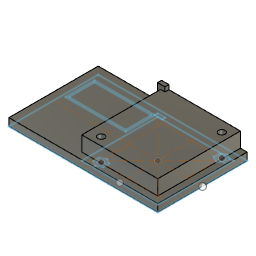
5015_TestBench v1 (Autodesk Fusion 360 design; units mm, degrees)
Autodesk Fusion 360 part; units mm, degrees
sketch "Sketch1" plane through (0, 0, 0) normal (0, 0, 1) x (1, 0, 0)
  line L0 (124.9201, 72.5503) -> (24.9201, 72.5503)
  line L1 (24.9201, 72.5503) -> (24.9201, 12.5503)
  line L2 (24.9201, 12.5503) -> (124.9201, 12.5503)
  line L3 (124.9201, 12.5503) -> (124.9201, 72.5503)
  line L4 (124.9201, 42.5503) -> (24.9201, 42.5503) construction
  line L5 (74.9201, 72.5503) -> (74.9201, 12.5503) construction
  line L6 (120.4201, 68.0503) -> (69.4201, 68.0503)
  line L7 (69.4201, 68.0503) -> (69.4201, 17.0503)
  line L8 (69.4201, 17.0503) -> (120.4201, 17.0503)
  line L9 (120.4201, 17.0503) -> (120.4201, 68.0503)
  line L10 (120.4201, 68.0503) -> (69.4201, 17.0503) construction
  line L11 (69.4201, 68.0503) -> (120.4201, 17.0503) construction
  line L12 (114.9201, 42.5503) -> (114.9201, 68.0503) construction
  line L13 (114.9201, 65.5503) -> (69.4201, 65.5503) construction
  circle A0 centre (114.9201, 65.5503) radius 2.25
  line L14 (69.4201, 22.5503) -> (120.4201, 22.5503) construction
  line L15 (94.9201, 68.0503) -> (94.9201, 17) construction
  line L16 (76.9201, 17.0503) -> (76.9201, 42.5503) construction
  circle A1 centre (76.9201, 22.5503) radius 2.25
  line L17 (118.3201, 67.5133) -> (114.9201, 69.4763)
  line L18 (114.9201, 69.4763) -> (111.5201, 67.5133)
  line L19 (111.5201, 67.5133) -> (111.5201, 63.5873)
  line L20 (111.5201, 63.5873) -> (114.9201, 61.6243)
  line L21 (114.9201, 61.6243) -> (118.3201, 63.5873)
  line L22 (118.3201, 63.5873) -> (118.3201, 67.5133)
  line L23 (80.3201, 24.5133) -> (76.9201, 26.4763)
  line L24 (76.9201, 26.4763) -> (73.5201, 24.5133)
  line L25 (73.5201, 24.5133) -> (73.5201, 20.5873)
  line L26 (73.5201, 20.5873) -> (76.9201, 18.6243)
  line L27 (76.9201, 18.6243) -> (80.3201, 20.5873)
  line L28 (80.3201, 20.5873) -> (80.3201, 24.5133)
  line L29 (67.4201, 68.0503) -> (26.9201, 68.0503)
  line L30 (26.9201, 68.0503) -> (26.9201, 48.5503)
  line L31 (26.9201, 48.5503) -> (67.4201, 48.5503)
  line L32 (67.4201, 48.5503) -> (67.4201, 68.0503)
  line L33 (28.1201, 49.7503) -> (66.2201, 49.7503)
  line L34 (66.2201, 49.7503) -> (66.2201, 66.8503)
  line L35 (66.2201, 66.8503) -> (28.1201, 66.8503)
  line L36 (28.1201, 66.8503) -> (28.1201, 49.7503)
  line L37 (67.4201, 68.0503) -> (72.4201, 68.0503)
  line L38 (72.4201, 68.0503) -> (72.4201, 70.0503)
  line L39 (72.4201, 70.0503) -> (67.4201, 70.0503)
  line L40 (67.4201, 70.0503) -> (67.4201, 68.0503)
  point P0 (94.9201, 42.5503)
  point P1 (114.9201, 65.5503)
  point P2 (76.9201, 22.5503)
  dimension "d1" = 100
  dimension "d2" = 60
  dimension "d3" = 51
  dimension "d4" = 51
  dimension "d5" = 45.5
  dimension "d6" = 23
  dimension "d7" = 4.5
  dimension "d8" = 20
  dimension "d10" = 18
  dimension "d11" = 4.5
  dimension "d18" = 3.4
  dimension "d19" = 3.4
  dimension "d22" = 19.5
  dimension "d23" = 2
  dimension "d24" = 2
  dimension "d25" = -1.2
  dimension "d26" = 5
  dimension "d27" = 2
  constraint horizontal L0
  constraint vertical L1
  constraint horizontal L2
  constraint vertical L3
  constraint midpoint L3 L4.start
  constraint midpoint L1 L4.end
  constraint midpoint L0 L5.start
  constraint midpoint L2 L5.end
  constraint horizontal L6
  constraint perpendicular L6 L7
  constraint parallel L6 L8
  constraint parallel L7 L9
  constraint coincident L10 P0
  constraint coincident L11 P0
  constraint coincident L4 P0
  constraint coincident L0.start L10
  constraint coincident L4 L12.start
  constraint coincident L6 L12.end
  constraint perpendicular L6 L12
  constraint coincident L12 P1
  constraint coincident L7 L13.end
  constraint perpendicular L7 L13
  constraint coincident P1 L13.start
  constraint coincident L7 L14.start
  constraint coincident L9 L14.end
  constraint perpendicular L9 L14
  constraint midpoint L6 L15.start
  constraint perpendicular L14 L15
  constraint coincident L8 L16.start
  constraint coincident L4 L16.end
  constraint perpendicular L4 L16
  constraint coincident L16 P2
  constraint coincident L14 P2
  constraint coincident P2 A1.centre
  constraint horizontal L29
  constraint vertical L30
  constraint horizontal L31
  constraint vertical L32
  constraint horizontal L37
  constraint vertical L38
  constraint horizontal L39
  constraint vertical L40
  measures "d1" distance of L0.start L0.end
  measures "d2" distance of L0.start L2.end
  measures "d3" distance of L7.end L8.end
  measures "d4" distance of L6.end L7.end
  measures "d5" distance of L7 L12
  measures "d6" distance of L4 L13
  measures "d7" diameter of A0
  measures "d8" distance of L4 L14
  measures "d10" distance of L15 L16
  measures "d11" diameter of A1
  measures "d18" distance of P1 L22
  measures "d19" distance of P2 L28
  measures "d22" distance of L29.start L31.end
  measures "d23" distance of L1 L30
  measures "d24" distance of L7 L32
  measures "d26" distance of L29.start L37.end
  measures "d27" distance of L29.start L39.end
extrude "Extrude1" add sketch "Sketch1" along normal blind 5 contours L0 L1 L2 L3 | L29 L30 L31 L32 | L6 L37 L38 L39 L40 | L6 L17 L18 | L33 L34 L35 L36
extrude "Extrude2" add sketch "Sketch1" along normal blind 15 contours L6 L7 L8 L9 L17 L18 L19 L20 L21 L22 L37 | L6 L17 L18 L19 L20 L21 L22 | L23 L24 L25 L26 L27 L28
extrude "Extrude3" add 1 faces at (103.4201, 68.0503, 8.3333) along direction (0, 1, 0) blind 4.5
extrude "Extrude4" cut sketch "Sketch1" along normal blind 3 contours L6 L17 L18 | L6 L17 L18 L19 L20 L21 L22 | L23 L24 L25 L26 L27 L28
extrude "Extrude5" add sketch "Sketch1" along normal blind 18 contours L6 L37 L38 L39 L40
sketch "Sketch2" plane through (0, 0, 0) normal (0, 0, 1) x (1, 0, 0)
extrude "Extrude6" cut 1 faces at (69.7535, 68.0503, 17) along direction (0, 1, 0) blind 1.8
extrude "Extrude7" add 1 faces at (69.7535, 70.0503, 17) along direction (0, 1, 0) blind 2.5
named bodies: "Support"
